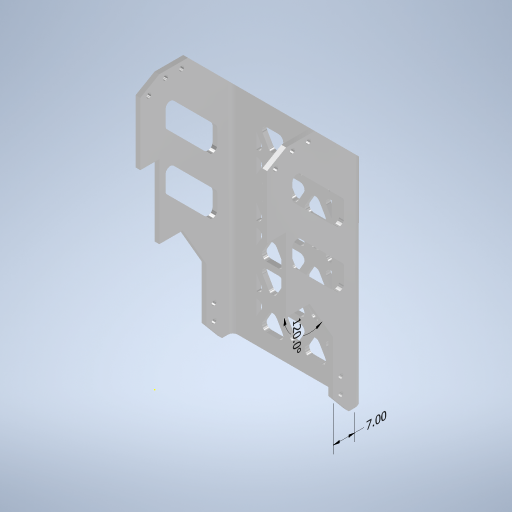
# Autodesk Inventor part: side
Saved by Autodesk Inventor 2024.1 (Build 281209000, 209)
## iProperties
Created: 2024-10-11
Part Number: side
Material: アルミニウム 6061
Document SubType Name: Sheet Metal
Designer: hibik
Density: 2.7 g/cm^3
Sheet Metal Rule: Default_mm
Appearance: アルミニウム - フラット
Author: hibik
Autodesk Inventor part; units mm, degrees
ref_plane "YZ Plane" through (0, 0, 0) normal (1, 0, 0) x (0, 1, 0)
ref_plane "XZ Plane" through (0, 0, 0) normal (0, 1, 0) x (-1, 0, 0)
ref_plane "XY Plane" through (0, 0, 0) normal (0, 0, 1) x (1, 0, 0)
sketch "スケッチ1" plane through (0, 0, 0) normal (1, 0, 0) x (0, 1, 0)
  line L0 (0, 0) -> (85, 0)
  line L1 (85, 0) -> (85, -20)
  line L2 (85, -20) -> (0, -20)
  line L3 (0, -20) -> (0, 0)
  circle A0 centre (0, -20) radius 1.6
  line L4 (-4, 0) -> (85, 0)
  line L5 (85, 0) -> (85, -25)
  line L6 (85, -25) -> (-4, -25)
  line L7 (-4, -25) -> (-4, 0)
  line L8 (-23, 0) -> (103, 0)
  line L9 (11, 0) -> (11, -15)
  line L10 (11, -15) -> (-0.9175, -25)
  line L11 (11, -15) -> (28.0096, -15)
  line L12 (28.0096, -15) -> (41, -7.5)
  line L13 (41, -7.5) -> (41, 0)
  circle A1 centre (0, -20) radius 5
  point P0 (4.9999, -20.0347)
  point P1 (0, -25)
  dimension "d0" = 85
  dimension "d1" = 20
  dimension "d2" = 3.2
  dimension "d3" = 4
  dimension "d4" = 5
  dimension "d5" = 5
  dimension "d6" = 11
  dimension "d7" = 50
  dimension "d8" = 7.5
  dimension "d9" = 120
  dimension "d10" = 41
  dimension "d11" = 15
  dimension "d12" = 10
  measures "d0" distance of L1.end L2.end
  measures "d1" distance of L2.end L0.start
  measures "d2" diameter of A0
  measures "d3" distance between parallel lines of L3 L7
  measures "d4" distance between parallel lines of L6 L2
  measures "d5" vertical distance of L9.end L2.end
  measures "d6" distance from line of L9 A0.centre
  measures "d7" angle of L9 L10
  measures "d8" distance of L12.end L13.end
  measures "d9" angle of L12 L13
  measures "d10" distance from line of L2.end L13
  measures "d11" distance between parallel lines of L0 L11
  measures "d12" diameter of A1
extrude "プレート1" add sketch "スケッチ1" along normal blind 1.5 contours L0 L1 L2 L10 L11 L12 L13 | L2 L5 L6 A1 L10
sketch "スケッチ2" plane through (1.5, 0, 0) normal (1, 0, 0) x (0, 0, -1)
  line L0 (2, 85) -> (2, 41)
  line L1 (0, 41) -> (0, 85) projected
  line L2 (7.5, 41) -> (0, 41) projected
  line L3 (0, 85) -> (25, 85) projected
  line L4 (2, 81) -> (18.5, 64.5)
  line L5 (18.5, 64.5) -> (18.5, 55.5)
  line L6 (18.5, 55.5) -> (2, 72)
  line L7 (2, 63) -> (18.5, 46.5)
  line L8 (18.5, 46.5) -> (18.5, 37.5)
  line L9 (18.5, 37.5) -> (2, 54)
  line L10 (25, 85) -> (25, 0) projected
  point P0 (0, 0)
  dimension "d14" = 2
  dimension "d15" = 135
  dimension "d16" = 9
  dimension "d17" = 6.5
  dimension "d18" = 9
  dimension "d19" = 13
  constraints: 14 end point, 5 point on line, 4 equal length, 2 collinear, 1 midpoint, 1 vertical
  measures "d14" distance between parallel lines of L1 L0
  measures "d15" angle of L0 L6
  measures "d16" distance of L4.end L5.end
  measures "d17" distance between parallel lines of L10 L5
  measures "d18" distance of L7.start L6.end
  measures "d19" distance from line of L2 L9.end
extrude "切り取り1" cut sketch "スケッチ2" against normal blind 1.5 contours L4 L5 L6 L0 | L7 L8 L9 L0
sketch "スケッチ3" plane through (1.5, 0, -23.5) normal (0, 0, -1) x (-1, 0, 0)
  line L0 (0, 85) -> (0, 0)
  line L1 (0, 0) -> (42, 0)
  line L2 (42, 0) -> (42, 85)
  line L3 (42, 85) -> (0, 85)
  constraints: 6 end point, 1 horizontal, 1 perpendicular, 1 vertical
edge flange "フランジ1" height 42 angle 90 thickness 1.5 bend radius 1.5 thickness toward (0, 0, -1) relief tear relief width 1.5 relief depth 0.75 edges at (0, 42.5, -25) wall of the first edge with corners at (1.5, 85, -23.5) (1.5, 0, -23.5) (-40.5, 0, -23.5) (-40.5, 85, -23.5)
bend "曲げ1"
corner "コーナー1"
sketch "スケッチ4" plane through (-39, 0, -25) normal (-1, 0, 0) x (0, -1, 0)
  line L0 (-85, 0) -> (0, 0)
  line L1 (0, 0) -> (0, 25)
  line L2 (0, 25) -> (-85, 25)
  line L3 (-85, 25) -> (-85, 0)
  constraints: 6 end point, 1 horizontal, 1 perpendicular, 1 vertical
edge flange "フランジ2" height 25 angle 90 thickness 1.5 bend radius 1.5 thickness toward (-1, 0, 0) relief tear relief width 1.5 relief depth 0.75 edges at (-40.5, 42.5, -23.5) wall of the first edge with corners at (-39, 85, -25) (-39, 0, -25) (-39, 0, 0) (-39, 85, 0)
bend "曲げ2"
corner "コーナー2"
sketch "スケッチ5" plane through (-39, 0, 0) normal (1, 0, 0) x (0, 0, -1)
  line L0 (22, 4.5826) -> (22, 85) projected
  line L1 (0, 85) -> (22, 85) projected
  line L2 (7.5, 41) -> (0, 41) projected
  line L3 (15, 28.0096) -> (7.5, 41) projected
  line L4 (15, 11) -> (15, 28.0096) projected
  line L5 (20.0347, 4.9999) -> (15, 11) projected
  arc A0 (22, 4.5826) -> (20.0347, 4.9999) centre (20, 0) ccw projected
  line L6 (18.5, 37.5) -> (2, 54) projected
  line L7 (2, 54) -> (2, 63) projected
  line L8 (2, 63) -> (18.5, 46.5) projected
  line L9 (18.5, 46.5) -> (18.5, 37.5) projected
  line L10 (2, 72) -> (2, 81) projected
  line L11 (22, 0) -> (22, 85) projected
  line L12 (22, 85) -> (0, 85) projected
  line L13 (0, 85) -> (0, 0) projected
  line L14 (22, 0) -> (0, 0) projected
  line L15 (2, 81) -> (18.5, 64.5) projected
  line L16 (18.5, 64.5) -> (18.5, 55.5) projected
  line L17 (18.5, 55.5) -> (2, 72) projected
  line L18 (0, 41) -> (0, 85) projected
  point P0 (0, 0)
  point P1 (0, 41)
  point P2 (22, 4.5826)
  point P3 (2, 85)
extrude "押し出し1" cut sketch "スケッチ5" against normal through all contours L11 L14 L13 L2 L3 L4 L5 A0 | L6 L7 L8 L9 | L10 L15 L16 L17
sketch "スケッチ7" plane through (-1.5, 0, -25) normal (0, 0, -1) x (-1, 0, 0)
  line L0 (0, 85) -> (36, 85) projected
  line L1 (6, 85) -> (30, 85)
  line L2 (30, 85) -> (30, 0)
  line L3 (30, 0) -> (6, 0)
  line L4 (6, 0) -> (6, 85)
  line L5 (0, 85) -> (0, 0) projected
  line L6 (36, 0) -> (36, 85) projected
  line L7 (6.6906, 67) -> (15.6906, 67) construction
  line L8 (15.6906, 67) -> (11.1906, 59.2058) construction
  line L9 (11.1906, 59.2058) -> (6.6906, 67) construction
  arc A0 (9.2887, 67) -> (7.9896, 64.75) centre (9.2887, 65.5) ccw
  arc A1 (14.3916, 64.75) -> (13.0925, 67) centre (13.0925, 65.5) ccw
  arc A2 (9.8916, 61.4558) -> (12.4896, 61.4558) centre (11.1906, 62.2058) ccw
  line L10 (18, 67) -> (13.5, 59.2058) construction
  line L11 (13.5, 59.2058) -> (22.5, 59.2058) construction
  line L12 (22.5, 59.2058) -> (18, 67) construction
  arc A3 (19.299, 64.75) -> (16.701, 64.75) centre (18, 64) ccw
  arc A4 (14.799, 61.4558) -> (16.0981, 59.2058) centre (16.0981, 60.7058) ccw
  arc A5 (19.9019, 59.2058) -> (21.201, 61.4558) centre (19.9019, 60.7058) ccw
  line L13 (9.2887, 67) -> (13.0925, 67)
  line L14 (14.3916, 64.75) -> (12.4896, 61.4558)
  line L15 (7.9896, 64.75) -> (9.8916, 61.4558)
  line L16 (16.701, 64.75) -> (14.799, 61.4558)
  line L17 (16.0981, 59.2058) -> (19.9019, 59.2058)
  line L18 (21.201, 61.4558) -> (19.299, 64.75)
  line L19 (20.3094, 67) -> (29.3094, 67) construction
  line L20 (29.3094, 67) -> (24.8094, 59.2058) construction
  line L21 (24.8094, 59.2058) -> (20.3094, 67) construction
  arc A6 (22.9075, 67) -> (21.6084, 64.75) centre (22.9075, 65.5) ccw
  arc A7 (28.0104, 64.75) -> (26.7113, 67) centre (26.7113, 65.5) ccw
  arc A8 (23.5104, 61.4558) -> (26.1084, 61.4558) centre (24.8094, 62.2058) ccw
  line L22 (22.9075, 67) -> (26.7113, 67)
  line L23 (28.0104, 64.75) -> (26.1084, 61.4558)
  line L24 (21.6084, 64.75) -> (23.5104, 61.4558)
  line L25 (6, 58.2058) -> (30, 58.2058) construction
  line L26 (6.6906, 49.4115) -> (15.6906, 49.4115) construction
  line L27 (15.6906, 49.4115) -> (11.1906, 57.2058) construction
  line L28 (11.1906, 57.2058) -> (6.6906, 49.4115) construction
  arc A9 (7.9896, 51.6615) -> (9.2887, 49.4115) centre (9.2887, 50.9115) ccw
  arc A10 (13.0925, 49.4115) -> (14.3916, 51.6615) centre (13.0925, 50.9115) ccw
  arc A11 (12.4896, 54.9558) -> (9.8916, 54.9558) centre (11.1906, 54.2058) ccw
  line L29 (18, 49.4115) -> (13.5, 57.2058) construction
  line L30 (13.5, 57.2058) -> (22.5, 57.2058) construction
  line L31 (22.5, 57.2058) -> (18, 49.4115) construction
  arc A12 (16.701, 51.6615) -> (19.299, 51.6615) centre (18, 52.4115) ccw
  arc A13 (16.0981, 57.2058) -> (14.799, 54.9558) centre (16.0981, 55.7058) ccw
  arc A14 (21.201, 54.9558) -> (19.9019, 57.2058) centre (19.9019, 55.7058) ccw
  line L32 (9.2887, 49.4115) -> (13.0925, 49.4115)
  line L33 (14.3916, 51.6615) -> (12.4896, 54.9558)
  line L34 (7.9896, 51.6615) -> (9.8916, 54.9558)
  line L35 (16.701, 51.6615) -> (14.799, 54.9558)
  line L36 (16.0981, 57.2058) -> (19.9019, 57.2058)
  line L37 (21.201, 54.9558) -> (19.299, 51.6615)
  line L38 (20.3094, 49.4115) -> (29.3094, 49.4115) construction
  line L39 (29.3094, 49.4115) -> (24.8094, 57.2058) construction
  line L40 (24.8094, 57.2058) -> (20.3094, 49.4115) construction
  arc A15 (21.6084, 51.6615) -> (22.9075, 49.4115) centre (22.9075, 50.9115) ccw
  arc A16 (26.7113, 49.4115) -> (28.0104, 51.6615) centre (26.7113, 50.9115) ccw
  line L41 (28.0104, 51.6615) -> (26.1084, 54.9558)
  arc A17 (26.1084, 54.9558) -> (23.5104, 54.9558) centre (24.8094, 54.2058) ccw
  line L42 (22.9075, 49.4115) -> (26.7113, 49.4115)
  line L43 (21.6084, 51.6615) -> (23.5104, 54.9558)
  arc A18 (5.6802, 64.75) -> (3.0822, 64.75) centre (4.3812, 64) ccw
  arc A19 (6.2831, 59.2058) -> (7.5822, 61.4558) centre (6.2831, 60.7058) ccw
  line L44 (7.5822, 61.4558) -> (5.6802, 64.75)
  line L45 (6.2831, 59.2058) -> (-10.927, 59.2058)
  arc A20 (32.9178, 64.75) -> (30.3198, 64.75) centre (31.6188, 64) ccw
  arc A21 (28.4178, 61.4558) -> (29.7169, 59.2058) centre (29.7169, 60.7058) ccw
  line L46 (30.3198, 64.75) -> (28.4178, 61.4558)
  line L47 (29.7169, 59.2058) -> (30, 59.2058)
  line L48 (7.5822, 54.9558) -> (5.6802, 51.6615)
  arc A22 (3.0822, 51.6615) -> (5.6802, 51.6615) centre (4.3812, 52.4115) ccw
  arc A23 (7.5822, 54.9558) -> (6.2831, 57.2058) centre (6.2831, 55.7058) ccw
  line L49 (6.2831, 57.2058) -> (-10.927, 57.2058)
  line L50 (30.3198, 51.6615) -> (28.4178, 54.9558)
  arc A24 (30.3198, 51.6615) -> (32.9178, 51.6615) centre (31.6188, 52.4115) ccw
  arc A25 (29.7169, 57.2058) -> (28.4178, 54.9558) centre (29.7169, 55.7058) ccw
  line L51 (29.7169, 57.2058) -> (30, 57.2058)
  line L52 (6.6906, 47.4115) -> (15.6906, 47.4115) construction
  line L53 (15.6906, 47.4115) -> (11.1906, 39.6173) construction
  arc A26 (9.8916, 41.8673) -> (12.4896, 41.8673) centre (11.1906, 42.6173) ccw
  line L54 (9.2887, 47.4115) -> (13.0925, 47.4115)
  line L55 (14.3916, 45.1615) -> (12.4896, 41.8673)
  arc A27 (14.3916, 45.1615) -> (13.0925, 47.4115) centre (13.0925, 45.9115) ccw
  arc A28 (14.799, 41.8673) -> (16.0981, 39.6173) centre (16.0981, 41.1173) ccw
  line L56 (16.701, 45.1615) -> (14.799, 41.8673)
  arc A29 (19.299, 45.1615) -> (16.701, 45.1615) centre (18, 44.4115) ccw
  line L57 (18, 47.4115) -> (13.5, 39.6173) construction
  arc A30 (28.4178, 41.8673) -> (29.7169, 39.6173) centre (29.7169, 41.1173) ccw
  line L58 (30.3198, 45.1615) -> (28.4178, 41.8673)
  arc A31 (32.9178, 45.1615) -> (30.3198, 45.1615) centre (31.6188, 44.4115) ccw
  line L59 (29.7169, 39.6173) -> (30, 39.6173)
  line L60 (22.5, 39.6173) -> (18, 47.4115) construction
  arc A32 (19.9019, 39.6173) -> (21.201, 41.8673) centre (19.9019, 41.1173) ccw
  line L61 (28.0104, 45.1615) -> (26.1084, 41.8673)
  arc A33 (23.5104, 41.8673) -> (26.1084, 41.8673) centre (24.8094, 42.6173) ccw
  arc A34 (28.0104, 45.1615) -> (26.7113, 47.4115) centre (26.7113, 45.9115) ccw
  line L62 (29.3094, 47.4115) -> (24.8094, 39.6173) construction
  line L63 (22.9075, 47.4115) -> (26.7113, 47.4115)
  line L64 (20.3094, 47.4115) -> (29.3094, 47.4115) construction
  line L65 (21.6084, 45.1615) -> (23.5104, 41.8673)
  line L66 (24.8094, 39.6173) -> (20.3094, 47.4115) construction
  line L67 (21.201, 41.8673) -> (19.299, 45.1615)
  arc A35 (22.9075, 47.4115) -> (21.6084, 45.1615) centre (22.9075, 45.9115) ccw
  arc A36 (21.201, 35.3673) -> (19.9019, 37.6173) centre (19.9019, 36.1173) ccw
  line L68 (21.201, 35.3673) -> (19.299, 32.0731)
  line L69 (22.5, 37.6173) -> (18, 29.8231) construction
  arc A37 (16.701, 32.0731) -> (19.299, 32.0731) centre (18, 32.8231) ccw
  line L70 (16.0981, 37.6173) -> (19.9019, 37.6173)
  line L71 (13.5, 37.6173) -> (22.5, 37.6173) construction
  line L72 (16.701, 32.0731) -> (14.799, 35.3673)
  line L73 (18, 29.8231) -> (13.5, 37.6173) construction
  arc A38 (16.0981, 37.6173) -> (14.799, 35.3673) centre (16.0981, 36.1173) ccw
  line L74 (6.6906, 29.8231) -> (15.6906, 29.8231) construction
  line L75 (15.6906, 29.8231) -> (11.1906, 37.6173) construction
  line L76 (11.1906, 37.6173) -> (6.6906, 29.8231) construction
  arc A39 (7.9896, 32.0731) -> (9.2887, 29.8231) centre (9.2887, 31.3231) ccw
  line L77 (6.2831, 37.6173) -> (-10.927, 37.6173)
  arc A40 (7.5822, 35.3673) -> (6.2831, 37.6173) centre (6.2831, 36.1173) ccw
  arc A41 (3.0822, 32.0731) -> (5.6802, 32.0731) centre (4.3812, 32.8231) ccw
  line L78 (7.5822, 35.3673) -> (5.6802, 32.0731)
  arc A42 (12.4896, 35.3673) -> (9.8916, 35.3673) centre (11.1906, 34.6173) ccw
  line L79 (7.9896, 32.0731) -> (9.8916, 35.3673)
  line L80 (14.3916, 32.0731) -> (12.4896, 35.3673)
  line L81 (9.2887, 29.8231) -> (13.0925, 29.8231)
  arc A43 (13.0925, 29.8231) -> (14.3916, 32.0731) centre (13.0925, 31.3231) ccw
  line L82 (13.5, 39.6173) -> (22.5, 39.6173) construction
  line L83 (16.0981, 39.6173) -> (19.9019, 39.6173)
  line L84 (6, 38.6173) -> (30, 38.6173) construction
  line L85 (28.0104, 32.0731) -> (26.1084, 35.3673)
  line L86 (29.3094, 29.8231) -> (24.8094, 37.6173) construction
  arc A44 (26.7113, 29.8231) -> (28.0104, 32.0731) centre (26.7113, 31.3231) ccw
  arc A45 (26.1084, 35.3673) -> (23.5104, 35.3673) centre (24.8094, 34.6173) ccw
  line L87 (21.6084, 32.0731) -> (23.5104, 35.3673)
  arc A46 (21.6084, 32.0731) -> (22.9075, 29.8231) centre (22.9075, 31.3231) ccw
  line L88 (24.8094, 37.6173) -> (20.3094, 29.8231) construction
  line L89 (22.9075, 29.8231) -> (26.7113, 29.8231)
  arc A47 (29.7169, 37.6173) -> (28.4178, 35.3673) centre (29.7169, 36.1173) ccw
  line L90 (20.3094, 29.8231) -> (29.3094, 29.8231) construction
  line L91 (30.3198, 32.0731) -> (28.4178, 35.3673)
  line L92 (29.7169, 37.6173) -> (30, 37.6173)
  arc A48 (30.3198, 32.0731) -> (32.9178, 32.0731) centre (31.6188, 32.8231) ccw
  line L93 (11.1906, 39.6173) -> (6.6906, 47.4115) construction
  arc A49 (9.2887, 47.4115) -> (7.9896, 45.1615) centre (9.2887, 45.9115) ccw
  line L94 (7.9896, 45.1615) -> (9.8916, 41.8673)
  arc A50 (6.2831, 39.6173) -> (7.5822, 41.8673) centre (6.2831, 41.1173) ccw
  line L95 (7.5822, 41.8673) -> (5.6802, 45.1615)
  arc A51 (5.6802, 45.1615) -> (3.0822, 45.1615) centre (4.3812, 44.4115) ccw
  line L96 (6.2831, 39.6173) -> (-10.927, 39.6173)
  line L97 (6.6906, 27.8231) -> (15.6906, 27.8231) construction
  line L98 (15.6906, 27.8231) -> (11.1906, 20.0289) construction
  arc A52 (9.8916, 22.2789) -> (12.4896, 22.2789) centre (11.1906, 23.0289) ccw
  line L99 (9.2887, 27.8231) -> (13.0925, 27.8231)
  line L100 (14.3916, 25.5731) -> (12.4896, 22.2789)
  arc A53 (14.3916, 25.5731) -> (13.0925, 27.8231) centre (13.0925, 26.3231) ccw
  arc A54 (14.799, 22.2789) -> (16.0981, 20.0289) centre (16.0981, 21.5289) ccw
  line L101 (16.701, 25.5731) -> (14.799, 22.2789)
  arc A55 (19.299, 25.5731) -> (16.701, 25.5731) centre (18, 24.8231) ccw
  line L102 (18, 27.8231) -> (13.5, 20.0289) construction
  arc A56 (28.4178, 22.2789) -> (29.7169, 20.0289) centre (29.7169, 21.5289) ccw
  line L103 (30.3198, 25.5731) -> (28.4178, 22.2789)
  arc A57 (32.9178, 25.5731) -> (30.3198, 25.5731) centre (31.6188, 24.8231) ccw
  line L104 (29.7169, 20.0289) -> (30, 20.0289)
  line L105 (22.5, 20.0289) -> (18, 27.8231) construction
  arc A58 (19.9019, 20.0289) -> (21.201, 22.2789) centre (19.9019, 21.5289) ccw
  line L106 (28.0104, 25.5731) -> (26.1084, 22.2789)
  arc A59 (23.5104, 22.2789) -> (26.1084, 22.2789) centre (24.8094, 23.0289) ccw
  arc A60 (28.0104, 25.5731) -> (26.7113, 27.8231) centre (26.7113, 26.3231) ccw
  line L107 (29.3094, 27.8231) -> (24.8094, 20.0289) construction
  line L108 (22.9075, 27.8231) -> (26.7113, 27.8231)
  line L109 (20.3094, 27.8231) -> (29.3094, 27.8231) construction
  line L110 (21.6084, 25.5731) -> (23.5104, 22.2789)
  line L111 (24.8094, 20.0289) -> (20.3094, 27.8231) construction
  line L112 (21.201, 22.2789) -> (19.299, 25.5731)
  arc A61 (22.9075, 27.8231) -> (21.6084, 25.5731) centre (22.9075, 26.3231) ccw
  arc A62 (21.201, 15.7789) -> (19.9019, 18.0289) centre (19.9019, 16.5289) ccw
  line L113 (21.201, 15.7789) -> (19.299, 12.4846)
  line L114 (22.5, 18.0289) -> (18, 10.2346) construction
  arc A63 (16.701, 12.4846) -> (19.299, 12.4846) centre (18, 13.2346) ccw
  line L115 (16.0981, 18.0289) -> (19.9019, 18.0289)
  line L116 (13.5, 18.0289) -> (22.5, 18.0289) construction
  line L117 (16.701, 12.4846) -> (14.799, 15.7789)
  line L118 (18, 10.2346) -> (13.5, 18.0289) construction
  arc A64 (16.0981, 18.0289) -> (14.799, 15.7789) centre (16.0981, 16.5289) ccw
  line L119 (6.6906, 10.2346) -> (15.6906, 10.2346) construction
  line L120 (15.6906, 10.2346) -> (11.1906, 18.0289) construction
  line L121 (11.1906, 18.0289) -> (6.6906, 10.2346) construction
  arc A65 (7.9896, 12.4846) -> (9.2887, 10.2346) centre (9.2887, 11.7346) ccw
  line L122 (6.2831, 18.0289) -> (-10.927, 18.0289)
  arc A66 (7.5822, 15.7789) -> (6.2831, 18.0289) centre (6.2831, 16.5289) ccw
  arc A67 (3.0822, 12.4846) -> (5.6802, 12.4846) centre (4.3812, 13.2346) ccw
  line L123 (7.5822, 15.7789) -> (5.6802, 12.4846)
  arc A68 (12.4896, 15.7789) -> (9.8916, 15.7789) centre (11.1906, 15.0289) ccw
  line L124 (7.9896, 12.4846) -> (9.8916, 15.7789)
  line L125 (14.3916, 12.4846) -> (12.4896, 15.7789)
  line L126 (9.2887, 10.2346) -> (13.0925, 10.2346)
  arc A69 (13.0925, 10.2346) -> (14.3916, 12.4846) centre (13.0925, 11.7346) ccw
  line L127 (13.5, 20.0289) -> (22.5, 20.0289) construction
  line L128 (16.0981, 20.0289) -> (19.9019, 20.0289)
  line L129 (6, 19.0289) -> (30, 19.0289) construction
  line L130 (28.0104, 12.4846) -> (26.1084, 15.7789)
  line L131 (29.3094, 10.2346) -> (24.8094, 18.0289) construction
  arc A70 (26.7113, 10.2346) -> (28.0104, 12.4846) centre (26.7113, 11.7346) ccw
  arc A71 (26.1084, 15.7789) -> (23.5104, 15.7789) centre (24.8094, 15.0289) ccw
  line L132 (21.6084, 12.4846) -> (23.5104, 15.7789)
  arc A72 (21.6084, 12.4846) -> (22.9075, 10.2346) centre (22.9075, 11.7346) ccw
  line L133 (24.8094, 18.0289) -> (20.3094, 10.2346) construction
  line L134 (22.9075, 10.2346) -> (26.7113, 10.2346)
  arc A73 (29.7169, 18.0289) -> (28.4178, 15.7789) centre (29.7169, 16.5289) ccw
  line L135 (20.3094, 10.2346) -> (29.3094, 10.2346) construction
  line L136 (30.3198, 12.4846) -> (28.4178, 15.7789)
  line L137 (29.7169, 18.0289) -> (30, 18.0289)
  arc A74 (30.3198, 12.4846) -> (32.9178, 12.4846) centre (31.6188, 13.2346) ccw
  line L138 (11.1906, 20.0289) -> (6.6906, 27.8231) construction
  arc A75 (9.2887, 27.8231) -> (7.9896, 25.5731) centre (9.2887, 26.3231) ccw
  line L139 (7.9896, 25.5731) -> (9.8916, 22.2789)
  arc A76 (6.2831, 20.0289) -> (7.5822, 22.2789) centre (6.2831, 21.5289) ccw
  line L140 (7.5822, 22.2789) -> (5.6802, 25.5731)
  arc A77 (5.6802, 25.5731) -> (3.0822, 25.5731) centre (4.3812, 24.8231) ccw
  line L141 (6.2831, 20.0289) -> (-10.927, 20.0289)
  line L142 (6.6906, 8.2346) -> (15.6906, 8.2346) construction
  line L143 (15.6906, 8.2346) -> (11.1906, 0.4404) construction
  arc A78 (9.8916, 2.6904) -> (12.4896, 2.6904) centre (11.1906, 3.4404) ccw
  line L144 (9.2887, 8.2346) -> (13.0925, 8.2346)
  line L145 (14.3916, 5.9846) -> (12.4896, 2.6904)
  arc A79 (14.3916, 5.9846) -> (13.0925, 8.2346) centre (13.0925, 6.7346) ccw
  arc A80 (14.799, 2.6904) -> (16.0981, 0.4404) centre (16.0981, 1.9404) ccw
  line L146 (16.701, 5.9846) -> (14.799, 2.6904)
  arc A81 (19.299, 5.9846) -> (16.701, 5.9846) centre (18, 5.2346) ccw
  line L147 (18, 8.2346) -> (13.5, 0.4404) construction
  arc A82 (28.4178, 2.6904) -> (29.7169, 0.4404) centre (29.7169, 1.9404) ccw
  line L148 (30.3198, 5.9846) -> (28.4178, 2.6904)
  arc A83 (32.9178, 5.9846) -> (30.3198, 5.9846) centre (31.6188, 5.2346) ccw
  line L149 (29.7169, 0.4404) -> (30, 0.4404)
  line L150 (22.5, 0.4404) -> (18, 8.2346) construction
  arc A84 (19.9019, 0.4404) -> (21.201, 2.6904) centre (19.9019, 1.9404) ccw
  line L151 (28.0104, 5.9846) -> (26.1084, 2.6904)
  arc A85 (23.5104, 2.6904) -> (26.1084, 2.6904) centre (24.8094, 3.4404) ccw
  arc A86 (28.0104, 5.9846) -> (26.7113, 8.2346) centre (26.7113, 6.7346) ccw
  line L152 (29.3094, 8.2346) -> (24.8094, 0.4404) construction
  line L153 (22.9075, 8.2346) -> (26.7113, 8.2346)
  line L154 (20.3094, 8.2346) -> (29.3094, 8.2346) construction
  line L155 (21.6084, 5.9846) -> (23.5104, 2.6904)
  line L156 (24.8094, 0.4404) -> (20.3094, 8.2346) construction
  line L157 (21.201, 2.6904) -> (19.299, 5.9846)
  arc A87 (22.9075, 8.2346) -> (21.6084, 5.9846) centre (22.9075, 6.7346) ccw
  arc A88 (21.201, -3.8096) -> (19.9019, -1.5596) centre (19.9019, -3.0596) ccw
  line L158 (21.201, -3.8096) -> (19.299, -7.1038)
  line L159 (22.5, -1.5596) -> (18, -9.3538) construction
  arc A89 (16.701, -7.1038) -> (19.299, -7.1038) centre (18, -6.3538) ccw
  line L160 (16.0981, -1.5596) -> (19.9019, -1.5596)
  line L161 (13.5, -1.5596) -> (22.5, -1.5596) construction
  line L162 (16.701, -7.1038) -> (14.799, -3.8096)
  line L163 (18, -9.3538) -> (13.5, -1.5596) construction
  arc A90 (16.0981, -1.5596) -> (14.799, -3.8096) centre (16.0981, -3.0596) ccw
  line L164 (6.6906, -9.3538) -> (15.6906, -9.3538) construction
  line L165 (15.6906, -9.3538) -> (11.1906, -1.5596) construction
  line L166 (11.1906, -1.5596) -> (6.6906, -9.3538) construction
  arc A91 (7.9896, -7.1038) -> (9.2887, -9.3538) centre (9.2887, -7.8538) ccw
  line L167 (6.2831, -1.5596) -> (-10.927, -1.5596)
  arc A92 (7.5822, -3.8096) -> (6.2831, -1.5596) centre (6.2831, -3.0596) ccw
  arc A93 (3.0822, -7.1038) -> (5.6802, -7.1038) centre (4.3812, -6.3538) ccw
  line L168 (7.5822, -3.8096) -> (5.6802, -7.1038)
  arc A94 (12.4896, -3.8096) -> (9.8916, -3.8096) centre (11.1906, -4.5596) ccw
  line L169 (7.9896, -7.1038) -> (9.8916, -3.8096)
  line L170 (14.3916, -7.1038) -> (12.4896, -3.8096)
  line L171 (9.2887, -9.3538) -> (13.0925, -9.3538)
  arc A95 (13.0925, -9.3538) -> (14.3916, -7.1038) centre (13.0925, -7.8538) ccw
  line L172 (13.5, 0.4404) -> (22.5, 0.4404) construction
  line L173 (16.0981, 0.4404) -> (19.9019, 0.4404)
  line L174 (6, -0.5596) -> (30, -0.5596) construction
  line L175 (28.0104, -7.1038) -> (26.1084, -3.8096)
  line L176 (29.3094, -9.3538) -> (24.8094, -1.5596) construction
  arc A96 (26.7113, -9.3538) -> (28.0104, -7.1038) centre (26.7113, -7.8538) ccw
  arc A97 (26.1084, -3.8096) -> (23.5104, -3.8096) centre (24.8094, -4.5596) ccw
  line L177 (21.6084, -7.1038) -> (23.5104, -3.8096)
  arc A98 (21.6084, -7.1038) -> (22.9075, -9.3538) centre (22.9075, -7.8538) ccw
  line L178 (24.8094, -1.5596) -> (20.3094, -9.3538) construction
  line L179 (22.9075, -9.3538) -> (26.7113, -9.3538)
  arc A99 (29.7169, -1.5596) -> (28.4178, -3.8096) centre (29.7169, -3.0596) ccw
  line L180 (20.3094, -9.3538) -> (29.3094, -9.3538) construction
  line L181 (30.3198, -7.1038) -> (28.4178, -3.8096)
  line L182 (29.7169, -1.5596) -> (30, -1.5596)
  arc A100 (30.3198, -7.1038) -> (32.9178, -7.1038) centre (31.6188, -6.3538) ccw
  line L183 (11.1906, 0.4404) -> (6.6906, 8.2346) construction
  arc A101 (9.2887, 8.2346) -> (7.9896, 5.9846) centre (9.2887, 6.7346) ccw
  line L184 (7.9896, 5.9846) -> (9.8916, 2.6904)
  arc A102 (6.2831, 0.4404) -> (7.5822, 2.6904) centre (6.2831, 1.9404) ccw
  line L185 (7.5822, 2.6904) -> (5.6802, 5.9846)
  arc A103 (5.6802, 5.9846) -> (3.0822, 5.9846) centre (4.3812, 5.2346) ccw
  line L186 (6.2831, 0.4404) -> (-10.927, 0.4404)
  line L187 (6.6906, -11.3538) -> (15.6906, -11.3538) construction
  line L188 (15.6906, -11.3538) -> (11.1906, -19.1481) construction
  arc A104 (9.8916, -16.8981) -> (12.4896, -16.8981) centre (11.1906, -16.1481) ccw
  line L189 (9.2887, -11.3538) -> (13.0925, -11.3538)
  line L190 (14.3916, -13.6038) -> (12.4896, -16.8981)
  arc A105 (14.3916, -13.6038) -> (13.0925, -11.3538) centre (13.0925, -12.8538) ccw
  arc A106 (14.799, -16.8981) -> (16.0981, -19.1481) centre (16.0981, -17.6481) ccw
  line L191 (16.701, -13.6038) -> (14.799, -16.8981)
  arc A107 (19.299, -13.6038) -> (16.701, -13.6038) centre (18, -14.3538) ccw
  line L192 (18, -11.3538) -> (13.5, -19.1481) construction
  arc A108 (28.4178, -16.8981) -> (29.7169, -19.1481) centre (29.7169, -17.6481) ccw
  line L193 (30.3198, -13.6038) -> (28.4178, -16.8981)
  arc A109 (32.9178, -13.6038) -> (30.3198, -13.6038) centre (31.6188, -14.3538) ccw
  line L194 (29.7169, -19.1481) -> (30, -19.1481)
  line L195 (22.5, -19.1481) -> (18, -11.3538) construction
  arc A110 (19.9019, -19.1481) -> (21.201, -16.8981) centre (19.9019, -17.6481) ccw
  line L196 (28.0104, -13.6038) -> (26.1084, -16.8981)
  arc A111 (23.5104, -16.8981) -> (26.1084, -16.8981) centre (24.8094, -16.1481) ccw
  arc A112 (28.0104, -13.6038) -> (26.7113, -11.3538) centre (26.7113, -12.8538) ccw
  line L197 (29.3094, -11.3538) -> (24.8094, -19.1481) construction
  line L198 (22.9075, -11.3538) -> (26.7113, -11.3538)
  line L199 (20.3094, -11.3538) -> (29.3094, -11.3538) construction
  line L200 (21.6084, -13.6038) -> (23.5104, -16.8981)
  line L201 (24.8094, -19.1481) -> (20.3094, -11.3538) construction
  line L202 (21.201, -16.8981) -> (19.299, -13.6038)
  arc A113 (22.9075, -11.3538) -> (21.6084, -13.6038) centre (22.9075, -12.8538) ccw
  arc A114 (21.201, -23.3981) -> (19.9019, -21.1481) centre (19.9019, -22.6481) ccw
  line L203 (21.201, -23.3981) -> (19.299, -26.6923)
  line L204 (22.5, -21.1481) -> (18, -28.9423) construction
  arc A115 (16.701, -26.6923) -> (19.299, -26.6923) centre (18, -25.9423) ccw
  line L205 (16.0981, -21.1481) -> (19.9019, -21.1481)
  line L206 (13.5, -21.1481) -> (22.5, -21.1481) construction
  line L207 (16.701, -26.6923) -> (14.799, -23.3981)
  line L208 (18, -28.9423) -> (13.5, -21.1481) construction
  arc A116 (16.0981, -21.1481) -> (14.799, -23.3981) centre (16.0981, -22.6481) ccw
  line L209 (6.6906, -28.9423) -> (15.6906, -28.9423) construction
  line L210 (15.6906, -28.9423) -> (11.1906, -21.1481) construction
  line L211 (11.1906, -21.1481) -> (6.6906, -28.9423) construction
  arc A117 (7.9896, -26.6923) -> (9.2887, -28.9423) centre (9.2887, -27.4423) ccw
  line L212 (6.2831, -21.1481) -> (-10.927, -21.1481)
  arc A118 (7.5822, -23.3981) -> (6.2831, -21.1481) centre (6.2831, -22.6481) ccw
  arc A119 (3.0822, -26.6923) -> (5.6802, -26.6923) centre (4.3812, -25.9423) ccw
  line L213 (7.5822, -23.3981) -> (5.6802, -26.6923)
  arc A120 (12.4896, -23.3981) -> (9.8916, -23.3981) centre (11.1906, -24.1481) ccw
  line L214 (7.9896, -26.6923) -> (9.8916, -23.3981)
  line L215 (14.3916, -26.6923) -> (12.4896, -23.3981)
  line L216 (9.2887, -28.9423) -> (13.0925, -28.9423)
  arc A121 (13.0925, -28.9423) -> (14.3916, -26.6923) centre (13.0925, -27.4423) ccw
  line L217 (13.5, -19.1481) -> (22.5, -19.1481) construction
  line L218 (16.0981, -19.1481) -> (19.9019, -19.1481)
  line L219 (6, -20.1481) -> (30, -20.1481) construction
  line L220 (28.0104, -26.6923) -> (26.1084, -23.3981)
  line L221 (29.3094, -28.9423) -> (24.8094, -21.1481) construction
  arc A122 (26.7113, -28.9423) -> (28.0104, -26.6923) centre (26.7113, -27.4423) ccw
  arc A123 (26.1084, -23.3981) -> (23.5104, -23.3981) centre (24.8094, -24.1481) ccw
  line L222 (21.6084, -26.6923) -> (23.5104, -23.3981)
  arc A124 (21.6084, -26.6923) -> (22.9075, -28.9423) centre (22.9075, -27.4423) ccw
  line L223 (24.8094, -21.1481) -> (20.3094, -28.9423) construction
  line L224 (22.9075, -28.9423) -> (26.7113, -28.9423)
  arc A125 (29.7169, -21.1481) -> (28.4178, -23.3981) centre (29.7169, -22.6481) ccw
  line L225 (20.3094, -28.9423) -> (29.3094, -28.9423) construction
  line L226 (30.3198, -26.6923) -> (28.4178, -23.3981)
  line L227 (29.7169, -21.1481) -> (30, -21.1481)
  arc A126 (30.3198, -26.6923) -> (32.9178, -26.6923) centre (31.6188, -25.9423) ccw
  line L228 (11.1906, -19.1481) -> (6.6906, -11.3538) construction
  arc A127 (9.2887, -11.3538) -> (7.9896, -13.6038) centre (9.2887, -12.8538) ccw
  line L229 (7.9896, -13.6038) -> (9.8916, -16.8981)
  arc A128 (6.2831, -19.1481) -> (7.5822, -16.8981) centre (6.2831, -17.6481) ccw
  line L230 (7.5822, -16.8981) -> (5.6802, -13.6038)
  arc A129 (5.6802, -13.6038) -> (3.0822, -13.6038) centre (4.3812, -14.3538) ccw
  line L231 (6.2831, -19.1481) -> (-10.927, -19.1481)
  line L232 (5.6802, 5.9846) -> (7.5822, 2.6904)
  arc A130 (6, 0.4674) -> (7.5822, 2.6904) centre (6.2831, 1.9404) ccw
  line L233 (6.2831, 0.4404) -> (4.7831, 0.4404)
  point P0 (-1.5, 0)
  point P1 (18, 85)
  point P2 (18, 65.4115)
  point P3 (6, 65.4115)
  point P4 (30, 65.4115)
  point P5 (18, 45.8231)
  point P6 (6, 45.8231)
  point P7 (30, 45.8231)
  point P8 (18, 26.2346)
  point P9 (6, 26.2346)
  point P10 (30, 26.2346)
  point P11 (18, 6.6462)
  point P12 (6, 6.6462)
  point P13 (30, 6.6462)
  point P14 (27.0333, 0)
  point P15 (22.5855, 0)
  point P16 (13.4145, 0)
  point P17 (8.9667, 0)
  point P18 (6, 12.1415)
  point P19 (6, 5.8519)
  point P20 (33, 17.1509)
  point P21 (30, 1.4404)
  point P22 (30, 5.8519)
  point P23 (33, 12.1415)
  point P24 (6, 31.7299)
  point P25 (6, 0.4404)
  point P26 (6, 1.4404)
  point P27 (6, 17.1509)
  point P28 (33, 36.7393)
  point P29 (30, 18.0289)
  point P30 (30, 0.4404)
  point P31 (33, 31.7299)
  point P32 (6, 18.0289)
  point P33 (6, 36.7393)
  point P34 (20.2761, 0)
  point P35 (15.7239, 0)
  point P36 (6, 51.3184)
  point P37 (6, 20.0289)
  point P38 (33, 56.3278)
  point P39 (30, 37.6173)
  point P40 (30, 20.0289)
  point P41 (33, 51.3184)
  point P42 (6, 70.9068)
  point P43 (6, 39.6173)
  point P44 (6, 37.6173)
  point P45 (6, 56.3278)
  point P46 (6, 57.2058)
  point P47 (6, 75.9163)
  point P48 (30, 39.6173)
  point P49 (33, 70.9068)
  point P50 (33, 75.9163)
  point P51 (30, 65.2058)
  point P52 (33, 90.4953)
  point P53 (6, 90.4953)
  point P54 (6, 59.2058)
  point P55 (6, 0.8423)
  point P56 (30, 8.45)
  point P57 (30, 0.8423)
  point P58 (6, 5.4308)
  point P59 (6, 8.45)
  point P60 (30, 13.0385)
  point P61 (30, 5.4308)
  point P62 (6, 13.0385)
  point P63 (6, 25.0192)
  point P64 (30, 32.6269)
  point P65 (30, 25.0192)
  point P66 (6, 44.6077)
  point P67 (6, 32.6269)
  point P68 (6, 52.2154)
  point P69 (30, 44.6077)
  point P70 (30, 52.2154)
  point P71 (30, 64.1962)
  point P72 (6, 64.1962)
  point P73 (29.5137, 0)
  point P74 (6.4863, 0)
  point P75 (27.2043, 0)
  point P76 (22.4145, 0)
  point P77 (20.1051, 0)
  point P78 (15.8949, 0)
  point P79 (13.5855, 0)
  point P80 (8.7957, 0)
  point P81 (6.2831, 0.4404)
  point P82 (6.3175, 0)
  point P83 (19.9363, 0)
  point P84 (16.0637, 0)
  point P85 (27.3731, 0)
  point P86 (22.2457, 0)
  point P87 (13.7543, 0)
  point P88 (8.6269, 0)
  point P89 (21.4007, 0)
  point P90 (14.5993, 0)
  point P91 (6.2831, 0.4404)
  dimension "d44" = 6
  dimension "d45" = 6
  dimension "d46" = 9
  dimension "d47" = 3
  dimension "d52" = 2
  dimension "d53" = 18
  dimension "d54" = 9
  dimension "d55" = 3
  dimension "d56" = 2
  dimension "d60" = 1
  dimension "d70" = 2
  dimension "d71" = 2
  dimension "d74" = 19.5885
  constraints: 456 end point, 421 vertical alignment, 263 point on circle, 212 point on line, 181 parallel, 131 centre point, 115 equal radius, 50 symmetric about line, 28 tangent, 9 equal length, 9 horizontal, 8 collinear, 1 coincident, 1 midpoint, 26 other
  measures "d46" distance of L7.start L7.end
  measures "d47" diameter of A0
  measures "d52" distance between parallel lines of L10 L8
  measures "d53" distance between parallel lines of L1 L7
  measures "d54" distance of L19.start L19.end
  measures "d55" diameter of A6
  measures "d56" distance between parallel lines of L12 L21
  measures "d60" distance between parallel lines of L11 L25
  measures "d70" distance between parallel lines of L15 L44
  measures "d71" distance between parallel lines of L20 L46
  measures "d74" distance of L7.start L52.start
extrude "押し出し2" cut sketch "スケッチ7" against normal through all contours L44 A19 L45 L4 | L2 L47 A21 L46 | L49 A23 L48 L4 | L4 L95 A50 L96 | L2 L50 A25 L51 | L77 A40 L78 L4 | L4 L140 A76 L141 | L2 L59 A30 L58 | L122 A66 L123 L4 | L2 L91 A47 L92 | L4 A130 L186 | L2 L104 A56 L103 | L2 L136 A73 L137 | L13 A1 L14 A2 L15 A0 | L18 A5 L17 A4 L16 A3 | L22 A7 L23 A8 L24 A6 | L34 A11 L33 A10 L32 A9 | L35 A13 L36 A14 L37 A12 | L43 A17 L41 A16 L42 A15 | L94 A49 L54 A27 L55 A26 | L56 A29 L67 A32 L83 A28 | L61 A33 L65 A35 L63 A34 | L68 A37 L72 A38 L70 A36 | L79 A42 L80 A43 L81 A39 | A44 L89 A46 L87 A45 L85 | L139 A75 L99 A53 L100 A52 | L101 A55 L112 A58 L128 A54 | L106 A59 L110 A61 L108 A60 | L113 A63 L117 A64 L115 A62 | L124 A68 L125 A69 L126 A65 | A70 L134 A72 L132 A71 L130 | L158 A89 L162 A90 L160 A88 | L169 A94 L170 A95 L171 A91 | A96 L179 A98 L177 A97 L175 | L229 A127 L189 A105 L190 A104 | L191 A107 L202 A110 L218 A106 | L196 A111 L200 A113 L198 A112 | L203 A115 L207 A116 L205 A114 | L214 A120 L215 A121 L216 A117 | A122 L224 A124 L222 A123 L220
fillet "フィレット1" radius 1.5 16 edges at (0.75, 81, -2) (0.75, 64.5, -18.5) (0.75, 55.5, -18.5) (0.75, 72, -2) (0.75, 63, -2) (0.75, 54, -2) (0.75, 37.5, -18.5) (0.75, 46.5, -18.5) (-39.75, 46.5, -18.5) (-39.75, 37.5, -18.5) (-39.75, 54, -2) (-39.75, 63, -2) (-39.75, 55.5, -18.5) (-39.75, 64.5, -18.5) (-39.75, 81, -2) (-39.75, 72, -2)
sketch "スケッチ9" plane through (1.5, 0, 0) normal (1, 0, 0) x (0, 0, -1)
  circle A0 centre (17.5, 16) radius 0.8 projected
  circle A1 centre (17.5, 11) radius 0.8 projected
  point P0 (0, 0)
extrude "押し出し3" cut sketch "スケッチ9" against normal through all
sketch "スケッチ10" plane through (-1.5, 0, -25) normal (0, 0, -1) x (-1, 0, 0)
  line L0 (-1.5, 4.9999) -> (-3, 4.9999) projected
  line L1 (-3, 4.9999) -> (39, 4.9999)
  line L2 (39, 4.9999) -> (39, 0)
  line L3 (39, 0) -> (-3, 0)
  line L4 (-3, 0) -> (-3, 4.9999)
  line L5 (36, 0) -> (0, 0) projected
  line L6 (39, 85) -> (39, 4.5826) projected
  point P0 (-1.5, 0)
  point P1 (-1.5, 4.9999)
  constraints: 8 end point, 2 collinear, 2 parallel, 1 horizontal, 1 perpendicular
extrude "押し出し4" cut sketch "スケッチ10" against normal through all
sketch "スケッチ11" plane through (1.5, 0, 0) normal (1, 0, 0) x (0, 0, -1)
  line L0 (0, 97.1421) -> (25, 72.1421)
  line L1 (25, 85) -> (25, 4.9999) projected
  line L2 (4.5607, 78.4393) -> (18.0607, 64.9393) projected
  line L3 (0, 41) -> (0, 85) projected
  line L4 (9.1421, 88) -> (0, 88)
  line L5 (0, 88) -> (-6.0622, 84.5)
  line L6 (-6.0622, 84.5) -> (-6.0622, 64.5)
  line L7 (7.5, 41) -> (0, 41) projected
  line L8 (-6.0622, 64.5) -> (0, 64.5)
  line L9 (0, 85) -> (22, 85) projected
  line L10 (25, 85) -> (22, 85) projected
  point P0 (0, 0)
  point P1 (12.1421, 85)
  dimension "d95" = 10
  dimension "d96" = 23.5
  dimension "d97" = 30
  dimension "d98" = 20
  dimension "d100" = 3
  constraints: 10 end point, 5 point on line, 1 horizontal, 1 parallel, 1 perpendicular, 1 vertical
  measures "d95" distance between parallel lines of L0 L2
  measures "d96" distance from line of L6.end L7
  measures "d97" angle of L4 L5
  measures "d98" distance of L5.end L6.end
  measures "d100" distance between parallel lines of L9 L4
sheet face with bend "面2" sketch "スケッチ11" thickness 1.5 toward (-1, 0, 0) bend radius 1.5 contours L0 L9 L3 L8 L6 L5 L4
bend "曲げ3"
extrude "押し出し5" cut sketch "スケッチ11" against normal through all contours L9 L10 L1 L0
sketch "スケッチ12" plane through (-40.5, 41, 0) normal (-1, 0, 0) x (0, 0, 1)
  circle A0 centre (-17.5, -25) radius 0.8
  circle A1 centre (-17.5, -30) radius 0.8
  line L0 (-9.1421, 47) -> (-22, 34.1421)
  line L1 (-22, 34.1421) -> (-22, -36.0001)
  line L2 (-22, -36.0001) -> (-20.0347, -36.0001)
  line L3 (-15, -30) -> (-20.0347, -36.0001)
  line L4 (-15, -12.9904) -> (-15, -30)
  line L5 (-7.5, 0) -> (-15, -12.9904)
  line L6 (0, 0) -> (-7.5, 0)
  line L7 (0, 23.5) -> (0, 0)
  line L8 (6.0622, 23.5) -> (0, 23.5)
  line L9 (6.0622, 43.5) -> (6.0622, 23.5)
  line L10 (0, 47) -> (6.0622, 43.5)
  line L11 (-9.1421, 47) -> (0, 47)
  line L12 (-2.4393, 30.5607) -> (-15.9393, 17.0607)
  arc A2 (-18.5, 18.1213) -> (-15.9393, 17.0607) centre (-17, 18.1213) ccw
  line L13 (-18.5, 18.1213) -> (-18.5, 22.8787)
  arc A3 (-18.0607, 23.9393) -> (-18.5, 22.8787) centre (-17, 22.8787) ccw
  line L14 (-18.0607, 23.9393) -> (-4.5607, 37.4393)
  arc A4 (-2, 36.3787) -> (-4.5607, 37.4393) centre (-3.5, 36.3787) ccw
  line L15 (-2, 36.3787) -> (-2, 31.6213)
  arc A5 (-2.4393, 30.5607) -> (-2, 31.6213) centre (-3.5, 31.6213) ccw
  line L16 (-2.4393, 12.5607) -> (-15.9393, -0.9393)
  arc A6 (-18.5, 0.1213) -> (-15.9393, -0.9393) centre (-17, 0.1213) ccw
  line L17 (-18.5, 0.1213) -> (-18.5, 4.8787)
  arc A7 (-18.0607, 5.9393) -> (-18.5, 4.8787) centre (-17, 4.8787) ccw
  line L18 (-18.0607, 5.9393) -> (-4.5607, 19.4393)
  arc A8 (-2, 18.3787) -> (-4.5607, 19.4393) centre (-3.5, 18.3787) ccw
  line L19 (-2, 18.3787) -> (-2, 13.6213)
  arc A9 (-2.4393, 12.5607) -> (-2, 13.6213) centre (-3.5, 13.6213) ccw
  line L20 (-12.1421, 44) -> (-22, 34.1421)
  line L21 (-22, 34.1421) -> (-22, -36.0001)
  line L22 (-22, -36.0001) -> (-20.0347, -36.0001)
  line L23 (-20.0347, -36.0001) -> (-15, -30)
  line L24 (-15, -30) -> (-15, -12.9904)
  line L25 (-15, -12.9904) -> (-7.5, 0)
  line L26 (-7.5, 0) -> (0, 0)
  line L27 (0, 44) -> (0, 0)
  line L28 (-12.1421, 44) -> (0, 44)
  circle A10 centre (-17.5, -25) radius 0.8
  circle A11 centre (-17.5, -30) radius 0.8
  line L29 (-2, 18.3787) -> (-2, 13.6213)
  arc A12 (-2.4393, 12.5607) -> (-2, 13.6213) centre (-3.5, 13.6213) ccw
  line L30 (-2.4393, 12.5607) -> (-15.9393, -0.9393)
  arc A13 (-18.5, 0.1213) -> (-15.9393, -0.9393) centre (-17, 0.1213) ccw
  line L31 (-18.5, 0.1213) -> (-18.5, 4.8787)
  arc A14 (-18.0607, 5.9393) -> (-18.5, 4.8787) centre (-17, 4.8787) ccw
  line L32 (-18.0607, 5.9393) -> (-4.5607, 19.4393)
  arc A15 (-2, 18.3787) -> (-4.5607, 19.4393) centre (-3.5, 18.3787) ccw
  line L33 (-18.5, 18.1213) -> (-18.5, 22.8787)
  arc A16 (-18.0607, 23.9393) -> (-18.5, 22.8787) centre (-17, 22.8787) ccw
  line L34 (-18.0607, 23.9393) -> (-4.5607, 37.4393)
  arc A17 (-2, 36.3787) -> (-4.5607, 37.4393) centre (-3.5, 36.3787) ccw
  line L35 (-2, 36.3787) -> (-2, 31.6213)
  arc A18 (-2.4393, 30.5607) -> (-2, 31.6213) centre (-3.5, 31.6213) ccw
  line L36 (-2.4393, 30.5607) -> (-15.9393, 17.0607)
  arc A19 (-18.5, 18.1213) -> (-15.9393, 17.0607) centre (-17, 18.1213) ccw
  point P0 (0, -41)
  point P1 (0, 23.5)
sheet face with bend "面3" sketch "スケッチ12" thickness 1.5 toward (1, 0, 0) bend radius 1.5 contours L11 L10 L9 L8 L27 L28 L0
bend "曲げ4"
sketch "スケッチ13" plane through (-40.5, 11, -15) normal (-1, 0, 0) x (0, 0, 1)
  point P0 (15, -11)
sketch "スケッチ14" plane through (-40.5, 11, -15) normal (-1, 0, 0) x (0, 0, 1)
  circle A0 centre (7.8579, 75) radius 0.8 projected
  circle A1 centre (13, 75) radius 0.8 projected
  circle A2 centre (18.3301, 72.7679) radius 0.8 projected
  point P0 (15, -11)
extrude "押し出し6" cut sketch "スケッチ14" against normal through all
equation "\"d18\" = d16"
equation "\"d20\" = Thickness"
equation "\"d45\" = d44"
equation "\"d56\" = d52"
equation "\"d70\" = d52"
equation "\"d71\" = d70"
equation "\"d13\" = Thickness"
equation "\"d22\" = BendReliefWidth"
equation "\"d23\" = BendReliefDepth"
equation "\"d24\" = MinimumRemnant"
equation "\"d25\" = TransitionRadius"
equation "\"d28\" = BendRadius"
equation "\"d29\" = CornerReliefSize"
equation "\"d30\" = GapSize"
equation "\"d31\" = JacobiRadiusSize"
equation "\"d32\" = BendReliefWidth"
equation "\"d33\" = BendReliefDepth"
equation "\"d34\" = MinimumRemnant"
equation "\"d35\" = TransitionRadius"
equation "\"d38\" = BendRadius"
equation "\"d39\" = CornerReliefSize"
equation "\"d40\" = GapSize"
equation "\"d41\" = JacobiRadiusSize"
equation "\"BendRadius\" = Thickness"
equation "\"BendReliefWidth\" = Thickness"
equation "\"BendReliefDepth\" = 0.5 * Thickness"
equation "\"CornerReliefSize\" = 4 * Thickness"
equation "\"MinimumRemnant\" = 2 * Thickness"
equation "\"TransitionRadius\" = BendRadius"
equation "\"JacobiRadiusSize\" = BendRadius"
equation "\"Thickness\" = 1.5"
equation "\"GapSize\" = 1.5"
